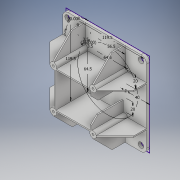
# Autodesk Inventor part: TurntableStand
Saved by Autodesk Inventor 2019.3 (Build 233278000, 278)
## iProperties
Created: 2019-07-07
Part Number: TurntableStand
Material: Generic
Document SubType Name: Modeling
Designer: mark
Density: 1 g/cm^3
Appearance: Default
Author: mark
Autodesk Inventor part; units mm, degrees
ref_plane "YZ Plane" through (0, 0, 0) normal (1, 0, 0) x (0, 1, 0)
ref_plane "XZ Plane" through (0, 0, 0) normal (0, 1, 0) x (-1, 0, 0)
ref_plane "XY Plane" through (0, 0, 0) normal (0, 0, 1) x (1, 0, 0)
sketch "BasePlate" plane through (0, 0, 0) normal (0, 0, 1) x (1, 0, 0)
  line L0 (56.5, 56.5) -> (0, 56.5)
  line L1 (0, 56.5) -> (0, 0)
  line L2 (0, 0) -> (56.5, 0)
  line L3 (56.5, 0) -> (56.5, 56.5)
  line L4 (96.5, 96.5) -> (-40, 96.5)
  line L5 (-40, 96.5) -> (-40, -40)
  line L6 (-40, -40) -> (96.5, -40)
  line L7 (96.5, -40) -> (96.5, 96.5)
  circle A0 centre (-4, 60.5) radius 1.75
  circle A1 centre (-4, 60.5) radius 5.25
  circle A2 centre (60.5, 60.5) radius 5.25
  circle A3 centre (60.5, 60.5) radius 1.75
  circle A4 centre (-4, -4) radius 5.25
  circle A5 centre (-4, -4) radius 1.75
  circle A6 centre (60.5, -4) radius 5.25
  circle A7 centre (60.5, -4) radius 1.75
  line L8 (58.5, 58.5) -> (-2, 58.5)
  line L9 (-2, 58.5) -> (-2, -2)
  line L10 (-2, -2) -> (58.5, -2)
  line L11 (58.5, -2) -> (58.5, 58.5)
  line L12 (56.5, 38.5) -> (58.5, 38.5)
  line L13 (56.5, 18) -> (58.5, 18)
  circle A8 centre (-32, 88.5) radius 4.5
  circle A9 centre (87.5, 88.5) radius 4.5
  circle A10 centre (-32, -31) radius 4.5
  circle A11 centre (87.5, -31) radius 4.5
  line L14 (-40, 61.5) -> (-9.1539, 61.5)
  line L15 (-9.1539, 61.5) -> (-9.1539, 59.5)
  line L16 (-9.1539, 59.5) -> (-40, 59.5)
  line L17 (-40, 59.5) -> (-40, 61.5)
  line L18 (-3, 96.5) -> (-3, 65.6539)
  line L19 (-5, 65.6539) -> (-5, 96.5)
  line L20 (-5, 96.5) -> (-3, 96.5)
  line L21 (-3, 65.6539) -> (-5, 65.6539)
  line L22 (0, 56.5) -> (56.5, 0)
  line L23 (56.5, 56.5) -> (0, 0)
  line L24 (-9.1539, -3) -> (-9.1539, -5)
  line L25 (-40, -5) -> (-40, -3)
  line L26 (-9.1539, -5) -> (-40, -5)
  line L27 (-40, -3) -> (-9.1539, -3)
  line L28 (-3, -9.1539) -> (-3, -40)
  line L29 (-5, -40) -> (-5, -9.1539)
  line L30 (-3, -40) -> (-5, -40)
  line L31 (-5, -9.1539) -> (-3, -9.1539)
  line L32 (59.5, -9.1539) -> (61.5, -9.1539)
  line L33 (61.5, -40) -> (59.5, -40)
  line L34 (61.5, -9.1539) -> (61.5, -40)
  line L35 (59.5, -40) -> (59.5, -9.1539)
  line L36 (65.6539, -3) -> (96.5, -3)
  line L37 (96.5, -5) -> (65.6539, -5)
  line L38 (96.5, -3) -> (96.5, -5)
  line L39 (65.6539, -5) -> (65.6539, -3)
  line L40 (65.6539, 59.5) -> (65.6539, 61.5)
  line L41 (96.5, 61.5) -> (96.5, 59.5)
  line L42 (65.6539, 61.5) -> (96.5, 61.5)
  line L43 (96.5, 59.5) -> (65.6539, 59.5)
  line L44 (59.5, 65.6539) -> (59.5, 96.5)
  line L45 (61.5, 96.5) -> (61.5, 65.6539)
  line L46 (59.5, 96.5) -> (61.5, 96.5)
  line L47 (61.5, 65.6539) -> (59.5, 65.6539)
  point P0 (28.25, 28.25)
  dimension "d0" = 56.5
  dimension "d102" = 40
  dimension "d104" = 3.5
  dimension "d105" = 3.5
  dimension "d106" = 4
  dimension "d107" = 4
  dimension "d110" = 64.5
  dimension "d113" = 64.5
  dimension "d116" = 2
  dimension "d117" = 20
  dimension "d118" = 20
  dimension "d119" = 9
  dimension "d120" = 8
  dimension "d121" = 8
  dimension "d124" = 119.5
  dimension "d127" = 119.5
  dimension "d130" = 2
  dimension "d133" = 90
  dimension "d137" = 360
  constraints: 96 end point, 12 centre point, 5 horizontal, 5 vertical, 4 point on line, 2 point on circle, 1 coincident, 1 collinear, 1 midpoint, 1 perpendicular, 95 other
  measures "d0" distance between parallel lines of L3 L1
  measures "d102" distance between parallel lines of L3 L7
  measures "d104" diameter of A0
  measures "d105" radial gap between concentric circles of A0 A1
  measures "d106" horizontal distance of A0.centre L0.end
  measures "d107" horizontal distance of A0.centre L0.end
  measures "d110" distance of A0.centre A2.centre
  measures "d113" distance of A0.centre A4.centre
  measures "d116" distance between parallel lines of L3 L11
  measures "d117" distance between parallel lines of L13 L10
  measures "d118" distance between parallel lines of L12 L8
  measures "d119" diameter of A8
  measures "d120" distance from line of L4 A8.centre
  measures "d121" distance from line of L5 A8.centre
  measures "d124" distance of A8.centre A9.centre
  measures "d127" distance of A8.centre A10.centre
  measures "d130" distance between parallel lines of L16 L14
extrude "Extrusion8" add sketch "BasePlate" along normal blind 5 contours L23 L22 L0 | L0 L1 L2 L3 L13 L11 A6 L10 A4 L9 A1 L8 A2 L12 | L3 L22 L23 | L22 L23 L1 | L12 L11 L13 L3 | L22 L2 L23 | L11 A2 L43 L7 L36 A6 | L11 L8 A2 L47 L40 | A2 L8 L11 | L11 L10 A6 | A6 L39 L32 L10 L11 | L8 A1 L18 L4 L44 A2 | L40 A2 | A2 L42 L7 L43 | L36 L7 L37 A6 | A6 L39 | A6 L35 L6 L28 A4 L10 | L44 L4 L45 A2 | A2 L47 | L8 L9 A1 L15 L21 | A1 L9 L8 | A2 L45 L4 L7 L42 | L37 L7 L6 L34 A6 | L32 A6 | A6 L34 L6 L35 | L10 L9 A4 | A4 L31 L24 L9 L10 | L9 A4 L27 L5 L16 A1 | L18 A1 L19 L4 | L16 L5 L14 A1 | A1 L15 | L21 A1 | L6 L29 A4 L28 | A4 L31 | L24 A4 | A4 L26 L5 L27 | L19 A1 L14 L5 L4 | L6 L5 L26 A4 L29 | A0 | A3 | A5 | A7
extrude "Extrusion9" add sketch "BasePlate" along normal blind 56.1 contours L0 L1 L2 L3 L13 L11 A6 L10 A4 L9 A1 L8 A2 L12 | L11 L8 A2 L47 L40 | A2 L8 L11 | L11 L10 A6 | A6 L39 L32 L10 L11 | L40 A2 | A2 L42 L7 L43 | L36 L7 L37 A6 | A6 L39 | L44 L4 L45 A2 | A2 L47 | L8 L9 A1 L15 L21 | A1 L9 L8 | L32 A6 | A6 L34 L6 L35 | L10 L9 A4 | A4 L31 L24 L9 L10 | L18 A1 L19 L4 | L16 L5 L14 A1 | A1 L15 | L21 A1 | L6 L29 A4 L28 | A4 L31 | L24 A4 | A4 L26 L5 L27
chamfer "Chamfer3" distance 10 angle 45 2 edges at (57.5, 18, 56.1) (57.5, 38.5, 56.1)
chamfer "Chamfer4" distance 30 angle 45 8 edges at (96.5, -4, 56.1) (60.5, -40, 56.1) (-4, -40, 56.1) (-40, -4, 56.1) (-40, 60.5, 56.1) (-4, 96.5, 56.1) (60.5, 96.5, 56.1) (96.5, 60.5, 56.1)
fillet "Fillet3" radius 9 4 edges at (96.5, -40, 2.5) (96.5, 96.5, 2.5) (-40, 96.5, 2.5) (-40, -40, 2.5)
body "Solid2"
